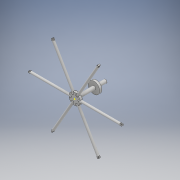
# Autodesk Inventor part: PropUp
Saved by Autodesk Inventor 2018 (Build 220112000, 112)
## iProperties
Created: 2019-06-02
Part Number: PropUp
Material: Generic
Document SubType Name: Modeling
Designer: dell
Density: 1 g/cm^3
Appearance: Default
Author: dell
Autodesk Inventor part; units mm, degrees
note: some values were not read from the file. Chosen so that the rebuilt part matches the saved one: copy form of "Circular Pattern3"; copy form of "Circular Pattern4".
ref_plane "XZ Plane" through (0, 0, 0) normal (0, 1, 0) x (-1, 0, 0)
sketch "Sketch1" plane through (0, 0, 0) normal (0, 1, 0) x (-1, 0, 0)
  circle A0 centre (0, 0) radius 50
  dimension "d0" = 100
  constraints: 1 centre point, 1 coincident
  measures "d0" diameter of A0
sketch "Sketch1 outline for Extrusion1" plane through (0, 0, 0) normal (0, 1, 0) x (-1, 0, 0)
  circle A0 centre (0, 0) radius 50
extrude "Extrusion1" add sketch "Sketch1 outline for Extrusion1" along normal blind 20
sketch "Sketch2" plane through (0, 20, 0) normal (0, 1, 0) x (1, 0, 0)
  line L0 (60.902375, 0) -> (39.097625, 0) construction
  circle A0 centre (0, 0) radius 50
  line L1 (60.902375, 10.5) -> (39.097625, 10.5)
  line L2 (39.097625, -10.5) -> (60.902375, -10.5)
  arc A1 (60.902375, -10.5) -> (60.902375, 10.5) centre (60.902375, 0) ccw
  arc A2 (39.097625, 10.5) -> (39.097625, -10.5) centre (39.097625, 0) ccw
  point P0 (50, 0)
  dimension "d4" = 21
  constraints: 8 end point, 4 point on circle, 4 tangent, 2 centre point, 1 horizontal, 1 horizontal alignment, 1 midpoint, 1 parallel, 1 other
  measures "d4" diameter of A2
sketch "Sketch2 outline for Extrusion2" plane through (0, 20, 0) normal (0, 1, 0) x (1, 0, 0)
  arc A0 (60.902375, -10.5) -> (60.902375, 10.5) centre (60.902375, 0) ccw
  line L0 (39.097625, -10.5) -> (60.902375, -10.5)
  arc A1 (39.097625, 10.5) -> (39.097625, -10.5) centre (39.097625, 0) ccw
  line L1 (60.902375, 10.5) -> (39.097625, 10.5)
extrude "Extrusion2" cut sketch "Sketch2 outline for Extrusion2" against normal blind 20
pattern_circular "Circular Pattern1" count 6 over 360 about axis through (0, -10, 0) along (0, 1, 0) of "Extrusion2"
sketch "Sketch3" plane through (0, 20, 0) normal (0, 1, 0) x (1, 0, 0)
  circle A0 centre (0, 0) radius 15
  dimension "d12" = 30
  constraints: 1 centre point, 1 coincident
  measures "d12" diameter of A0
sketch "Sketch3 outline for Extrusion3" plane through (0, 20, 0) normal (0, 1, 0) x (1, 0, 0)
  circle A0 centre (0, 0) radius 15
extrude "Extrusion3" add sketch "Sketch3 outline for Extrusion3" along normal blind 250
ref_plane "Work Plane2" through (0, 95, 0) normal (0, 1, 0) x (1, 0, 0)
mirror "Mirror1" about plane through (0, 95, 0) normal (0, 1, 0) of "Extrusion1"
ref_plane "Work Plane5" through (400, 0, 0) normal (1, 0, 0) x (0, 1, 0)
sketch "Sketch5" plane through (400, 0, 0) normal (1, 0, 0) x (0, 1, 0)
  line L0 (20, 10.5) -> (20, -10.5) projected
  line L1 (20, 10.5) -> (0, 10.5) projected
  line L2 (0, -10.5) -> (0, 10.5) projected
  line L3 (20, -10.5) -> (0, -10.5) projected
  circle A0 centre (10, 0) radius 10
  point P0 (0, 0)
  dimension "d20" = 20
  dimension "d21" = 10
  constraints: 1 centre point
  measures "d20" diameter of A0
  measures "d21" distance from line of L0 A0.centre
sketch "Sketch5 outline for Extrusion4" plane through (400, 0, 0) normal (1, 0, 0) x (0, 1, 0)
  circle A0 centre (10, 0) radius 10
extrude "Extrusion4" add sketch "Sketch5 outline for Extrusion4" against normal up to next
pattern_circular "Circular Pattern2" count 6 over 360 about axis through (0, -10, 0) along (0, 1, 0) of "Extrusion4"
sketch "Sketch6" plane through (400, 10, 0) normal (1, 0, 0) x (0, 0, -1)
  circle A0 centre (0, 0) radius 10
  point P0 (0, -10)
  constraints: 1 centre point
sketch "Sketch6 outline for Extrusion5" plane through (400, 10, 0) normal (1, 0, 0) x (0, 0, -1)
  circle A0 centre (0, 0) radius 10
extrude "Extrusion5" add sketch "Sketch6 outline for Extrusion5" along normal blind 10
pattern_circular "Circular Pattern3" count 6 over 360 about axis through (0, -10, 0) along (0, 1, 0) of "Extrusion4" geometry pattern yes
pattern_circular "Circular Pattern4" count 6 over 360 about axis through (0, -10, 0) along (0, 1, 0) of "Extrusion5", "Extrusion4" geometry pattern yes
sketch "Sketch7" plane through (0, 0, 0) normal (0, 1, 0) x (-1, 0, 0)
  point P0 (0, 0)
sketch "Sketch8" plane through (0, 0, 0) normal (0, 1, 0) x (-1, 0, 0)
  line L0 (-395, -5) -> (-425, -5)
  line L1 (-425, -5) -> (-425, 5)
  line L2 (-425, 5) -> (-395, 5)
  line L3 (-395, 5) -> (-395, -5)
  line L4 (-410, 10) -> (-410, -10)
  line L5 (-395, -5) -> (-425, 5) construction
  line L6 (-425, -5) -> (-395, 5) construction
  line L7 (-395, 5) -> (-410, 5)
  line L8 (-410, 5) -> (-410, 10)
  line L9 (-410, 10) -> (-395, 10)
  line L10 (-395, 10) -> (-395, 5)
  line L11 (-410, -10) -> (-35.896063, -10)
  line L12 (-410, -5) -> (-395, -5)
  line L13 (-395, -5) -> (-395, -10)
  line L14 (-395, -10) -> (-410, -10)
  line L15 (-410, -10) -> (-410, -5)
  point P0 (0, 0)
  point P1 (-410, 0)
  dimension "d35" = 30
  dimension "d36" = 10
  constraints: 28 end point, 6 parallel, 4 midpoint, 3 horizontal, 3 perpendicular, 3 point on line
  measures "d35" distance of L1.end L2.end
  measures "d36" distance of L0.end L1.end
sketch "Sketch8 outline for Extrusion6" plane through (0, 0, 0) normal (0, 1, 0) x (-1, 0, 0)
  line L0 (-395, -5) -> (-410, -5)
  line L1 (-395, -10) -> (-395, -5)
  line L2 (-410, -10) -> (-395, -10)
  line L3 (-410, -5) -> (-410, -10)
  line L4 (-410, 5) -> (-395, 5)
  line L5 (-410, 10) -> (-410, 5)
  line L6 (-395, 10) -> (-410, 10)
  line L7 (-395, 5) -> (-395, 10)
extrude "Extrusion6" cut sketch "Sketch8 outline for Extrusion6" along normal blind 50
pattern_circular "Circular Pattern5" count 6 over 360 about axis through (0, -10, 0) along (0, 1, 0) of "Extrusion6"
sketch "Sketch9" plane through (395, 1.339746, 5) normal (0, 0, 1) x (1, 0, 0)
  circle A0 centre (8.099004, 8.627225) radius 5
  point P0 (-395, -1.339746)
  dimension "d42" = 10
  constraints: 1 centre point
  measures "d42" diameter of A0
sketch "Sketch9 outline for Extrusion7" plane through (395, 1.339746, 5) normal (0, 0, 1) x (1, 0, 0)
  circle A0 centre (8.099004, 8.627225) radius 5
extrude "Extrusion7" cut sketch "Sketch9 outline for Extrusion7" against normal blind 50
pattern_circular "Circular Pattern6" count 6 over 360 about axis through (0, -10, 0) along (0, 1, 0) of "Extrusion7"
body "Solid1"
